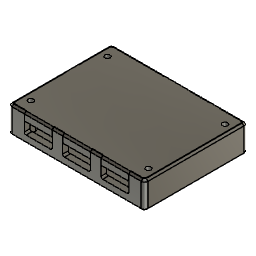
HDMI_Switcher v4 (Autodesk Fusion 360 design; units mm, degrees)
Autodesk Fusion 360 part; units mm, degrees
sketch "Sketch1" plane through (0, 0, 0) normal (0, 0, 1) x (1, 0, 0)
  line L0 (37, -29.5) -> (-37, -29.5)
  line L1 (-38.75, -27.5) -> (-38.75, 27.5)
  line L2 (-37, 29.5) -> (37, 29.5)
  line L3 (38.75, 27.5) -> (38.75, -27.5)
  line L4 (38.75, -29.5) -> (-38.75, 29.5) construction
  line L5 (-38.75, -29.5) -> (38.75, 29.5) construction
  line L6 (36, -28.5) -> (-36, -28.5)
  line L7 (-37.75, -26.5) -> (-37.75, 26.5)
  line L8 (-36, 28.5) -> (36, 28.5)
  line L9 (37.75, 26.5) -> (37.75, -26.5)
  line L10 (37.75, -28.5) -> (-37.75, 28.5) construction
  line L11 (-37.75, -28.5) -> (37.75, 28.5) construction
  arc A0 (-36.75, 29.5) -> (-38.75, 27.5) centre (-36.75, 27.5) ccw
  arc A1 (-35.75, 28.5) -> (-37.75, 26.5) centre (-35.75, 26.5) ccw
  arc A2 (38.75, 27.5) -> (36.75, 29.5) centre (36.75, 27.5) ccw
  arc A3 (37.75, 26.5) -> (35.75, 28.5) centre (35.75, 26.5) ccw
  arc A4 (36.75, -29.5) -> (38.75, -27.5) centre (36.75, -27.5) ccw
  arc A5 (35.75, -28.5) -> (37.75, -26.5) centre (35.75, -26.5) ccw
  arc A6 (-38.75, -27.5) -> (-36.75, -29.5) centre (-36.75, -27.5) ccw
  arc A7 (-37.75, -26.5) -> (-35.75, -28.5) centre (-35.75, -26.5) ccw
  line L12 (38.75, 26) -> (-38.75, 26)
  line L13 (-38.75, -26) -> (38.75, -26)
  line L14 (-38.75, 11.529) -> (-37.75, 11.2315) construction
  line L15 (37.75, -11.2315) -> (38.75, -11.529) construction
  line L16 (38.75, 11.529) -> (37.75, 11.2315) construction
  line L17 (-37.75, -11.2315) -> (-38.75, -11.529) construction
  line L18 (-37.75, 22.1895) -> (-33.75, 22.1895)
  line L19 (-33.75, 22.1895) -> (-33.75, -35)
  line L20 (-33.75, -26) -> (-33.75, -15)
  circle A8 centre (-33.75, -15) radius 2
  line L21 (-33.75, -15) -> (-33.75, -8.8)
  line L22 (-33.75, -15) -> (-33.75, -2)
  circle A9 centre (-33.75, -8.8) radius 2
  circle A10 centre (-33.75, -2) radius 2
  line L23 (-37.75, 24.2353) -> (-33.15, 24.2353)
  line L24 (-33.15, 24.2353) -> (-33.15, 26)
  line L25 (-33.15, 26) -> (-33.15, 15)
  circle A11 centre (-33.15, 15) radius 2
  line L26 (-33.75, 26) -> (-33.75, 22)
  circle A12 centre (-33.75, 22) radius 2.5
  line L27 (37.75, 26) -> (33.75, 26)
  line L28 (33.75, 26) -> (33.75, 22)
  line L29 (33.75, 22) -> (37.75, 22)
  line L30 (37.75, 22) -> (37.75, 26)
  circle A13 centre (33.75, 22) radius 2.5
  line L31 (37.75, -26) -> (33.75, -26)
  line L32 (33.75, -26) -> (33.75, -22)
  line L33 (33.75, -22) -> (37.75, -22)
  line L34 (37.75, -22) -> (37.75, -26)
  circle A14 centre (33.75, -22) radius 2.5
  line L35 (-37.75, -26) -> (-33.75, -26)
  line L36 (-33.75, -26) -> (-33.75, -22)
  line L37 (-33.75, -22) -> (-37.75, -22)
  line L38 (-37.75, -22) -> (-37.75, -26)
  circle A15 centre (-33.75, -22) radius 2.5
  line L39 (0, -26) -> (8, -26)
  line L40 (8, -26) -> (8, -29.5)
  line L41 (0, -26) -> (-8, -26)
  line L42 (-8, -26) -> (-8, -29.5)
  line L43 (0, 26) -> (8, 26)
  line L44 (8, 26) -> (8, 29.5)
  line L45 (0, 28.5) -> (-8, 28.5)
  line L46 (-8, 28.5) -> (-8, 29.5)
  line L47 (8, -26) -> (30, -26)
  line L48 (30, -26) -> (14, -26)
  line L49 (14, -26) -> (14, -29.5)
  line L50 (30, -26) -> (30, -29.5)
  line L51 (-8, -26) -> (-30, -26)
  line L52 (-30, -26) -> (-30, -29.5)
  line L53 (-30, -26) -> (-14, -26)
  line L54 (-14, -26) -> (-14, -29.5)
  line L55 (-39, -27.5) -> (-39, 27.5)
  arc A16 (-37, 29.5) -> (-39, 27.5) centre (-37, 27.5) ccw
  line L56 (-38, -26.5) -> (-38, 26.5)
  arc A17 (-36, 28.5) -> (-38, 26.5) centre (-36, 26.5) ccw
  arc A18 (-38, -26.5) -> (-36, -28.5) centre (-36, -26.5) ccw
  arc A19 (-39, -27.5) -> (-37, -29.5) centre (-37, -27.5) ccw
  line L57 (38, 26.5) -> (38, -26.5)
  line L58 (39, 27.5) -> (39, -27.5)
  arc A20 (38, 26.5) -> (36, 28.5) centre (36, 26.5) ccw
  arc A21 (39, 27.5) -> (37, 29.5) centre (37, 27.5) ccw
  arc A22 (36, -28.5) -> (38, -26.5) centre (36, -26.5) ccw
  arc A23 (37, -29.5) -> (39, -27.5) centre (37, -27.5) ccw
  line L59 (-8, 28.5) -> (-8, 26)
  line L60 (-8, 26) -> (-10, 26)
  line L61 (-10, 26) -> (-10, 26.25)
  line L62 (-10, 26.25) -> (-8, 26.25)
  line L63 (-10, 26.25) -> (-10, 28.5)
  line L64 (8, 26) -> (8, 26.25)
  line L65 (8, 26.25) -> (10, 26.25)
  line L66 (10, 26.25) -> (10, 28.5)
  line L67 (-8, -26) -> (-8, -26.25)
  line L68 (-8, -26.25) -> (-32, -26.25)
  line L69 (-32, -26.25) -> (31.5597, -26.25)
  line L70 (-30, -26.25) -> (-32, -26.25)
  line L71 (-32, -26.25) -> (-32, -28.5)
  line L72 (-14, -26.25) -> (-12, -26.25)
  line L73 (-12, -26.25) -> (-12, -28.5)
  line L74 (-8, -26.25) -> (-10, -26.25)
  line L75 (-10, -26.25) -> (-10, -28.5)
  line L76 (8, -26.25) -> (10, -26.25)
  line L77 (10, -26.25) -> (10, -28.5)
  line L78 (14, -26.25) -> (12, -26.25)
  line L79 (12, -26.25) -> (12, -28.5)
  line L80 (30, -26.25) -> (32, -26.25)
  line L81 (32, -26.25) -> (32, -28.5)
  line L82 (37.75, 26) -> (24.45, 26)
  line L83 (24.45, 26) -> (24.45, 28.5)
  line L84 (24.45, 28.5) -> (18.45, 28.5)
  line L85 (18.45, 28.5) -> (18.45, 29.5)
  line L86 (24.45, 28.5) -> (24.45, 29.5)
  line L87 (-38, 26) -> (-38, 10)
  line L88 (-38, 10) -> (-38, 2)
  line L89 (-38, 2) -> (-39, 2)
  line L90 (-38, 10) -> (-39, 10)
  circle A24 centre (-33.75, 22) radius 1.75
  circle A25 centre (-33.75, -22) radius 1.75
  circle A26 centre (33.75, 22) radius 1.75
  circle A27 centre (33.75, -22) radius 1.75
  line L91 (-37.5, -26.5) -> (-37.5, 26.5)
  arc A28 (-36, 28) -> (-37.5, 26.5) centre (-36, 26.5) ccw
  line L92 (-36, 28) -> (36, 28)
  arc A29 (37.5, 26.5) -> (36, 28) centre (36, 26.5) ccw
  line L93 (37.5, 26.5) -> (37.5, -26.5)
  arc A30 (36, -28) -> (37.5, -26.5) centre (36, -26.5) ccw
  line L94 (36, -28) -> (-36, -28)
  arc A31 (-37.5, -26.5) -> (-36, -28) centre (-36, -26.5) ccw
  line L95 (18.45, 28.5) -> (18.45, 28)
  line L96 (18.45, 28) -> (18.45, 26)
  line L97 (-32, -26.25) -> (-37.5, -26.25)
  line L98 (32, -26.25) -> (37.5, -26.25)
  line L99 (37.5, -26.25) -> (38, -26.25)
  line L100 (-37.5, -26.25) -> (-38, -26.25)
  line L101 (-78, -26.25) -> (-78, -28.5)
  line L102 (-90, 28.5) -> (-98, 28.5)
  line L103 (-126, 28.5) -> (-54, 28.5)
  line L104 (-100, 26.25) -> (-100, 28.5)
  line L105 (-100, 26) -> (-100, 26.25)
  line L106 (-82, 26.25) -> (-80, 26.25)
  line L107 (-71.55, 28.5) -> (-71.55, 29.5)
  line L108 (-104, -26.25) -> (-102, -26.25)
  arc A32 (-129, -27.5) -> (-127, -29.5) centre (-127, -27.5) ccw
  line L109 (-90, 26) -> (-82, 26)
  line L110 (-98, -26.25) -> (-122, -26.25)
  circle A33 centre (-123.75, -22) radius 2.5
  line L111 (-120, -26.25) -> (-122, -26.25)
  arc A34 (-52, 26.5) -> (-54, 28.5) centre (-54, 26.5) ccw
  arc A35 (-51, 27.5) -> (-53, 29.5) centre (-53, 27.5) ccw
  arc A36 (-128, -26.5) -> (-126, -28.5) centre (-126, -26.5) ccw
  line L112 (-65.55, 28.5) -> (-65.55, 29.5)
  line L113 (-104, -26) -> (-104, -29.5)
  line L114 (-71.55, 28.5) -> (-71.55, 28)
  line L115 (-128.75, 11.529) -> (-127.75, 11.2315) construction
  line L116 (-98, -26) -> (-98, -26.25)
  line L117 (-127.5, -26.25) -> (-128, -26.25)
  line L118 (-100, 26.25) -> (-98, 26.25)
  line L119 (-51.25, 11.529) -> (-52.25, 11.2315) construction
  arc A37 (-127, 29.5) -> (-129, 27.5) centre (-127, 27.5) ccw
  line L120 (-127.75, -22) -> (-127.75, -26)
  line L121 (-98, -26.25) -> (-100, -26.25)
  line L122 (-102, -26.25) -> (-102, -28.5)
  line L123 (-60, -26) -> (-60, -29.5)
  circle A38 centre (-56.25, -22) radius 2.5
  line L124 (-51.25, 26) -> (-128.75, 26)
  line L125 (-122, -26.25) -> (-127.5, -26.25)
  line L126 (-80, 26.25) -> (-80, 28.5)
  line L127 (-65.55, 26) -> (-65.55, 28.5)
  line L128 (-128, 10) -> (-129, 10)
  line L129 (-52.25, -22) -> (-52.25, -26)
  line L130 (-120, -26) -> (-120, -29.5)
  line L131 (-82, -26.25) -> (-80, -26.25)
  line L132 (-82, 26) -> (-82, 29.5)
  line L133 (-52.5, -26.25) -> (-52, -26.25)
  line L134 (-52.25, 26) -> (-65.55, 26)
  line L135 (-98, -26) -> (-98, -29.5)
  line L136 (-60, -26.25) -> (-58, -26.25)
  line L137 (-122, -26.25) -> (-122, -28.5)
  line L138 (-65.55, 28.5) -> (-71.55, 28.5)
  circle A39 centre (-56.25, 22) radius 2.5
  circle A40 centre (-56.25, 22) radius 1.75
  line L139 (-128, 2) -> (-129, 2)
  line L140 (-98, 28.5) -> (-98, 29.5)
  line L141 (-52.25, 26) -> (-56.25, 26)
  line L142 (-100, -26.25) -> (-100, -28.5)
  line L143 (-82, -26) -> (-82, -29.5)
  line L144 (-80, -26.25) -> (-80, -28.5)
  line L145 (-98, 26) -> (-100, 26)
  line L146 (-82, 26) -> (-82, 26.25)
  line L147 (-128, 10) -> (-128, 2)
  line L148 (-52.25, 22) -> (-52.25, 26)
  line L149 (-71.55, 28) -> (-71.55, 26)
  line L150 (-98, 28.5) -> (-98, 26)
  arc A41 (-126, 28.5) -> (-128, 26.5) centre (-126, 26.5) ccw
  circle A42 centre (-123.75, -22) radius 1.75
  line L151 (-128, 26) -> (-128, 10)
  line L152 (-58, -26.25) -> (-58, -28.5)
  circle A43 centre (-123.75, 22) radius 1.75
  circle A44 centre (-123.75, 22) radius 2.5
  arc A45 (-125.75, 28.5) -> (-127.0797, 27.9939) centre (-125.75, 26.5) ccw
  line L153 (-58, -26.25) -> (-52.5, -26.25)
  line L154 (-52, 26.5) -> (-52, -26.5)
  line L155 (-76, -26) -> (-76, -29.5)
  arc A46 (-54, -28.5) -> (-52, -26.5) centre (-54, -26.5) ccw
  line L156 (-122, -26.25) -> (-58.4403, -26.25)
  arc A47 (-53, -29.5) -> (-51, -27.5) centre (-53, -27.5) ccw
  line L157 (-76, -26.25) -> (-78, -26.25)
  circle A48 centre (-56.25, -22) radius 1.75
  line L158 (-51, 27.5) -> (-51, -27.5)
  line L159 (-52.25, -11.2315) -> (-51.25, -11.529) construction
  line L160 (-128, -26.5) -> (-128, 26.5)
  line L161 (-127, 29.5) -> (-98, 29.5)
  line L162 (-98, 29.5) -> (-82, 29.5)
  line L163 (-82, 29.5) -> (-71.55, 29.5)
  line L164 (-53.25, 29.5) -> (-53, 29.5)
  line L165 (-65.55, 29.5) -> (-53.25, 29.5)
  line L166 (-71.55, 29.5) -> (-65.55, 29.5)
  line L167 (-129, -27.5) -> (-129, 2)
  line L168 (-129, 10) -> (-129, 27.5)
  line L169 (-129, 2) -> (-129, 10)
  line L170 (-120, -29.5) -> (-127, -29.5)
  line L171 (-104, -29.5) -> (-120, -29.5)
  line L172 (-120, -28.5) -> (-126, -28.5)
  line L173 (-104, -28.5) -> (-120, -28.5)
  line L174 (-98, -29.5) -> (-104, -29.5)
  line L175 (-82, -29.5) -> (-98, -29.5)
  line L176 (-98, -28.5) -> (-104, -28.5)
  line L177 (-82, -28.5) -> (-98, -28.5)
  line L178 (-53, -29.5) -> (-60, -29.5)
  line L179 (-76, -29.5) -> (-82, -29.5)
  line L180 (-60, -29.5) -> (-76, -29.5)
  line L181 (-54, -28.5) -> (-60, -28.5)
  line L182 (-76, -28.5) -> (-82, -28.5)
  line L183 (-60, -28.5) -> (-76, -28.5)
  line L184 (-127.75, 24.2353) -> (-127.5, 24.2353)
  line L185 (-127.75, 22.1895) -> (-127.5, 22.1895)
  line L186 (-123.75, 22.1895) -> (-123.75, 22)
  line L187 (-123.75, 26) -> (-123.75, 25.4801)
  arc A49 (-126, 28.25) -> (-127.75, 26.5) centre (-126, 26.5) ccw
  line L188 (-127.75, -26.5) -> (-127.75, 26.5)
  arc A50 (-127.75, -26.5) -> (-126, -28.25) centre (-126, -26.5) ccw
  line L189 (-120, -28.25) -> (-126, -28.25)
  line L190 (-104, -28.25) -> (-120, -28.25)
  line L191 (-98, -28.25) -> (-104, -28.25)
  line L192 (-82, -28.25) -> (-98, -28.25)
  line L193 (-76, -28.25) -> (-82, -28.25)
  line L194 (-60, -28.25) -> (-76, -28.25)
  line L195 (-54, -28.25) -> (-60, -28.25)
  arc A51 (-54, -28.25) -> (-52.25, -26.5) centre (-54, -26.5) ccw
  line L196 (-52.25, 26.5) -> (-52.25, -26.5)
  arc A52 (-52.25, 26.5) -> (-54, 28.25) centre (-54, 26.5) ccw
  line L197 (-126, 28.25) -> (-54, 28.25)
  line L198 (-98, 26) -> (-97.9, 26)
  line L199 (-97.9, 26) -> (-97.9, 28.25)
  line L200 (-82, 26) -> (-82.1, 26)
  line L201 (-82.1, 26) -> (-82.1, 28.25)
  line L202 (-71.55, 26) -> (-71.45, 26)
  line L203 (-71.45, 26) -> (-71.45, 28.25)
  line L204 (-65.55, 26) -> (-65.65, 26)
  line L205 (-65.65, 26) -> (-65.65, 28.25)
  line L206 (-129, 10) -> (-129, 9.9)
  line L207 (-129, 9.9) -> (-127.75, 9.9)
  line L208 (-129, 2) -> (-129, 2.1)
  line L209 (-129, 2.1) -> (-127.75, 2.1)
  line L210 (-120, -26.25) -> (-119.9, -26.25)
  line L211 (-119.9, -26.25) -> (-119.9, -29.5)
  line L212 (-104, -29.5) -> (-104.1, -29.5)
  line L213 (-104.1, -29.5) -> (-104.0981, -26.25)
  line L214 (-98, -29.5) -> (-97.9, -29.5)
  line L215 (-97.9, -29.5) -> (-97.9, -26.25)
  line L216 (-82, -29.5) -> (-82.1, -29.5)
  line L217 (-82.1, -29.5) -> (-82.1, -26.25)
  line L218 (-76, -29.5) -> (-75.9, -29.5)
  line L219 (-75.9, -29.5) -> (-75.9, -26.25)
  line L220 (-60, -29.5) -> (-60.1, -29.5)
  line L221 (-60.1, -29.5) -> (-60.1, -26.25)
  line L222 (-97.9, 28.25) -> (-97.9, 29.5)
  line L223 (-82.1, 28.25) -> (-82.1, 29.5)
  line L224 (-71.45, 28.25) -> (-71.45, 29.5)
  line L225 (-65.65, 28.25) -> (-65.65, 29.5)
  line L226 (-33.75, 24.5) -> (-37.5, 24.5)
  line L227 (-33.75, 19.5) -> (-37.5, 19.5)
  line L228 (33.75, 24.5) -> (37.5, 24.5)
  line L229 (33.75, 19.5) -> (37.5, 19.5)
  line L230 (33.75, -24.5) -> (37.5, -24.5)
  line L231 (33.75, -19.5) -> (37.5, -19.5)
  line L232 (-33.75, -19.5) -> (-37.5, -19.5)
  line L233 (-33.75, -24.5) -> (-37.5, -24.5)
  line L234 (-31.25, 22) -> (-31.25, 26)
  line L235 (31.25, 22) -> (31.25, 26.5)
  line L236 (31.25, -22) -> (31.25, -27)
  line L237 (-31.25, -22) -> (-31.25, -27)
  circle A53 centre (-56.25, 22) radius 1.5
  circle A54 centre (-123.75, -22) radius 1.5
  circle A55 centre (-56.25, -22) radius 1.5
  circle A56 centre (-123.75, 22) radius 1.5
  line L238 (-38, 10) -> (-37.5, 10)
  line L239 (-38, 2) -> (-37.5, 2)
  point P0 (-90, 0)
  point P1 (-90, 0)
  point P2 (-90, 0)
  dimension "d1" = 77.5
  dimension "d2" = 59
  dimension "d3" = 75.5
  dimension "d4" = 57
  dimension "d5" = 2
  dimension "d6" = 2
  dimension "d8" = 4
  dimension "d9" = 11
  dimension "d10" = 4
  dimension "d11" = 6.2
  dimension "d12" = 13
  dimension "d13" = 4
  dimension "d14" = 4
  dimension "d15" = 4.6
  dimension "d16" = 11
  dimension "d17" = 4
  dimension "d19" = 4
  dimension "d20" = 5
  dimension "d21" = 4
  dimension "d22" = 4
  dimension "d23" = 5
  dimension "d24" = 4
  dimension "d25" = 4
  dimension "d26" = 5
  dimension "d27" = 4
  dimension "d28" = 4
  dimension "d29" = 5
  dimension "d32" = 8
  dimension "d33" = 8
  dimension "d34" = 8
  dimension "d35" = 8
  dimension "d36" = 22
  dimension "d37" = 16
  dimension "d38" = 22
  dimension "d39" = 16
  dimension "d41" = 2
  dimension "d43" = 2
  dimension "d46" = 2
  dimension "d47" = 2
  dimension "d48" = 0.25
  dimension "d49" = 0.25
  dimension "d50" = 2
  dimension "d51" = 0.25
  dimension "d52" = 2
  dimension "d53" = 2
  dimension "d54" = 2
  dimension "d55" = 2
  dimension "d56" = 2
  dimension "d57" = 2
  dimension "d58" = 13.3
  dimension "d59" = 6
  dimension "d62" = 16
  dimension "d63" = 8
  dimension "d72" = 3.5
  dimension "d73" = 3.5
  dimension "d74" = 3.5
  dimension "d75" = 3.5
  dimension "d80" = -0.5
  dimension "d102" = 4
  dimension "d103" = 4
  dimension "d104" = 5
  dimension "d106" = 4
  dimension "d107" = 5
  dimension "d109" = 4
  dimension "d110" = 5
  dimension "d113" = 8
  dimension "d114" = 8
  dimension "d115" = 22
  dimension "d116" = 16
  dimension "d117" = 22
  dimension "d118" = 16
  dimension "d124" = 2
  dimension "d126" = 2
  dimension "d127" = 0.25
  dimension "d128" = 0.25
  dimension "d129" = 2
  dimension "d130" = 0.25
  dimension "d131" = 2
  dimension "d132" = 2
  dimension "d133" = 2
  dimension "d134" = 2
  dimension "d135" = 2
  dimension "d136" = 2
  dimension "d137" = 13.3
  dimension "d138" = 6
  dimension "d139" = 16
  dimension "d140" = 8
  dimension "d142" = 3.5
  dimension "d143" = 3.5
  dimension "d144" = 3.5
  dimension "d145" = 0.25
  dimension "d146" = 0.1
  dimension "d147" = 0.1
  dimension "d148" = 0.1
  dimension "d149" = 0.1
  dimension "d150" = 0.1
  dimension "d151" = 0.1
  dimension "d152" = 0.1
  dimension "d153" = 0.1
  dimension "d154" = 0.1
  dimension "d155" = 0.1
  dimension "d156" = 0.1
  dimension "d157" = 0.1
  dimension "d174" = 3
  dimension "d176" = 3
  dimension "d177" = 3
  dimension "d178" = 3
  constraint horizontal L0
  constraint perpendicular L0 L1
  constraint parallel L0 L2
  constraint parallel L1 L3
  constraint coincident L4 origin
  constraint coincident L5 origin
  constraint horizontal L6
  constraint perpendicular L6 L7
  constraint parallel L6 L8
  constraint parallel L7 L9
  constraint coincident L10 origin
  constraint coincident L11 origin
  constraint coincident L4.end L1
  constraint coincident L4.end L2
  constraint tangent L1 A0
  constraint tangent L2 A0
  constraint coincident L10.end L8
  constraint coincident L10.end L7
  constraint tangent L8 A1
  constraint tangent L7 A1
  constraint coincident L5.end L2
  constraint coincident L5.end L3
  constraint tangent L2 A2
  constraint tangent L3 A2
  constraint equal A1 A2
  constraint coincident L11.end L8
  constraint coincident L11.end L9
  constraint tangent L8 A3
  constraint tangent L9 A3
  constraint equal A1 A3
  constraint coincident L4.start L0
  constraint coincident L4.start L3
  constraint tangent L0 A4
  constraint tangent L3 A4
  constraint equal A1 A4
  constraint coincident L10.start L9
  constraint coincident L10.start L6
  constraint tangent L9 A5
  constraint tangent L6 A5
  constraint equal A1 A5
  constraint coincident L5.start L0
  constraint coincident L5.start L1
  constraint tangent L0 A6
  constraint tangent L1 A6
  constraint equal A1 A6
  constraint coincident L11.start L7
  constraint coincident L11.start L6
  constraint tangent L7 A7
  constraint tangent L6 A7
  constraint equal A1 A7
  constraint horizontal L12
  constraint parallel L12 L13
  constraint coincident origin L16
  constraint coincident origin L14
  constraint coincident L1 L12.end
  constraint coincident L1 L13.start
  constraint coincident L1 L17.end
  constraint coincident L1 L14.start
  constraint coincident L3 L15.end
  constraint coincident L3 L16.start
  constraint coincident L3 L12.start
  constraint coincident L3 L13.end
  constraint coincident L9 L15.start
  constraint collinear L14 L15
  constraint coincident L9 L16.end
  constraint collinear L16 L17
  constraint coincident L7 L14.end
  constraint coincident L7 L17.start
  constraint coincident L7 L18.start
  constraint perpendicular L7 L18
  constraint perpendicular L0 L19
  constraint coincident L19 L20.start
  constraint coincident L13 L20.start
  constraint perpendicular L13 L20
  constraint coincident L20.end A8.centre
  constraint parallel L19 L21
  constraint parallel L21 L22
  constraint coincident L21.end A9.centre
  constraint coincident L22.end A10.centre
  constraint coincident L7 L23.start
  constraint perpendicular L7 L23
  constraint coincident L12 L24.end
  constraint perpendicular L12 L24
  constraint perpendicular L23 L25
  constraint coincident L25.end A11.centre
  constraint coincident L12 L26.start
  constraint perpendicular L23 L26
  constraint coincident L26.end A12.centre
  constraint horizontal L27
  constraint vertical L28
  constraint horizontal L29
  constraint vertical L30
  constraint coincident L9 L27.start
  constraint coincident L12 L27.start
  constraint coincident L28.end L29.start
  constraint horizontal L31
  constraint vertical L32
  constraint horizontal L33
  constraint vertical L34
  constraint coincident L9 L31.start
  constraint coincident L13 L31.start
  constraint coincident L32.end L33.start
  constraint horizontal L35
  constraint vertical L36
  constraint horizontal L37
  constraint vertical L38
  constraint coincident L7 L35.start
  constraint coincident L13 L35.start
  constraint coincident L36.end L37.start
  constraint midpoint L13 L39.start
  constraint parallel L13 L39
  constraint coincident L0 L40.end
  constraint perpendicular L0 L40
  constraint perpendicular L40 L41
  constraint coincident L0 L42.end
  constraint perpendicular L0 L42
  constraint midpoint L12 L43.start
  constraint perpendicular L3 L43
  constraint coincident L2 L44.end
  constraint perpendicular L2 L44
  constraint perpendicular L44 L45
  constraint coincident L2 L46.end
  constraint perpendicular L2 L46
  constraint perpendicular L40 L47
  constraint coincident L47 L48.end
  constraint coincident L0 L49.end
  constraint perpendicular L0 L49
  constraint coincident L0 L50.end
  constraint perpendicular L0 L50
  constraint perpendicular L42 L51
  constraint coincident L0 L52.end
  constraint perpendicular L0 L52
  constraint perpendicular L52 L53
  constraint coincident L0 L54.end
  constraint perpendicular L0 L54
  constraint coincident L2 A0.start
  constraint tangent L2 A16
  constraint tangent L55 A16
  constraint coincident L8 L45.start
  constraint coincident L8 A1.start
  constraint tangent L8 A17
  constraint tangent L56 A17
  constraint coincident L6 A7.end
  constraint tangent L6 A18
  constraint tangent L56 A18
  constraint equal A17 A18
  constraint coincident L0 A6.end
  constraint tangent L0 A19
  constraint tangent L55 A19
  constraint equal A17 A19
  constraint coincident L8 A3.end
  constraint tangent L8 A20
  constraint tangent L57 A20
  constraint coincident L2 A2.end
  constraint tangent L58 A21
  constraint tangent L2 A21
  constraint equal A20 A21
  constraint coincident L6 A5.start
  constraint tangent L57 A22
  constraint tangent L6 A22
  constraint equal A20 A22
  constraint coincident L0 A4.start
  constraint tangent L58 A23
  constraint tangent L0 A23
  constraint equal A20 A23
  constraint coincident L12 L59.end
  constraint perpendicular L12 L59
  constraint coincident L12 L60.end
  constraint perpendicular L60 L61
  constraint coincident L59 L62.end
  constraint perpendicular L59 L62
  constraint coincident L8 L63.end
  constraint perpendicular L8 L63
  constraint vertical L64
  constraint perpendicular L44 L65
  constraint coincident L8 L66.end
  constraint perpendicular L8 L66
  constraint vertical L67
  constraint perpendicular L52 L68
  constraint parallel L13 L69
  constraint coincident L52 L70.start
  constraint coincident L68 L70.start
  constraint perpendicular L52 L70
  constraint coincident L6 L71.end
  constraint perpendicular L6 L71
  constraint coincident L54 L72.start
  constraint coincident L68 L72.start
  constraint perpendicular L54 L72
  constraint coincident L6 L73.end
  constraint perpendicular L6 L73
  constraint perpendicular L42 L74
  constraint coincident L6 L75.end
  constraint perpendicular L6 L75
  constraint coincident L40 L76.start
  constraint coincident L69 L76.start
  constraint perpendicular L40 L76
  constraint coincident L6 L77.end
  constraint perpendicular L6 L77
  constraint coincident L49 L78.start
  constraint perpendicular L49 L78
  constraint coincident L6 L79.end
  constraint perpendicular L6 L79
  constraint coincident L50 L80.start
  constraint coincident L69 L80.start
  constraint perpendicular L50 L80
  constraint coincident L6 L81.end
  constraint perpendicular L6 L81
  constraint coincident L12 L82.end
  constraint coincident L8 L83.end
  constraint perpendicular L8 L83
  constraint coincident L8 L84.end
  constraint coincident L2 L85.end
  constraint perpendicular L2 L85
  constraint coincident L2 L86.end
  constraint perpendicular L2 L86
  constraint coincident L56 L87.start
  constraint coincident L12 L87.start
  constraint perpendicular L18 L87
  constraint parallel L7 L88
  constraint coincident L55 L89.end
  constraint perpendicular L55 L89
  constraint coincident L55 L90.end
  constraint perpendicular L55 L90
  constraint concentric A12 A24
  constraint concentric A15 A25
  constraint concentric A13 A26
  constraint concentric A14 A27
  constraint coincident L92 L95.end
  constraint perpendicular L92 L95
  constraint coincident L12 L96.end
  constraint perpendicular L12 L96
  constraint coincident L91 L97.end
  constraint perpendicular L91 L97
  constraint coincident L93 L98.end
  constraint perpendicular L93 L98
  constraint coincident L57 L99.end
  constraint perpendicular L57 L99
  constraint coincident L56 L100.end
  constraint perpendicular L56 L100
  constraint horizontal L178
  constraint parallel L161 L178
  constraint horizontal L181
  constraint parallel L103 L181
  constraint tangent L103 A45
  constraint horizontal L124
  constraint coincident P2 L119
  constraint coincident P2 L115
  constraint coincident P2 P1
  constraint collinear L115 L159
  constraint coincident L187.start L124
  constraint perpendicular L184 L187
  constraint coincident A43.centre A44.centre
  constraint horizontal L141
  constraint vertical L148
  constraint coincident L134.start L124
  constraint vertical L129
  constraint vertical L120
  constraint perpendicular L143 L178
  constraint coincident L135.end L178
  constraint perpendicular L135 L178
  constraint midpoint L109.start L124
  constraint coincident L132.end L161
  constraint perpendicular L132 L161
  constraint perpendicular L102 L132
  constraint perpendicular L140 L161
  constraint coincident L155.end L178
  constraint perpendicular L155 L178
  constraint perpendicular L123 L178
  constraint coincident L130.end L178
  constraint perpendicular L130 L178
  constraint perpendicular L113 L178
  constraint tangent A37 L161
  constraint tangent A37 L167
  constraint coincident L102.start L103
  constraint coincident A45.start L103
  constraint tangent L103 A41
  constraint tangent A41 L160
  constraint tangent A36 L181
  constraint tangent A36 L160
  constraint equal A36 A41
  constraint tangent A32 L178
  constraint tangent A32 L167
  constraint equal A32 A41
  constraint tangent L103 A34
  constraint tangent A34 L154
  constraint coincident L164.start L161
  constraint tangent A35 L158
  constraint tangent A35 L161
  constraint equal A34 A35
  constraint tangent L154 A46
  constraint tangent A46 L181
  constraint equal A34 A46
  constraint tangent A47 L158
  constraint tangent A47 L178
  constraint equal A34 A47
  constraint coincident L145.start L124
  constraint perpendicular L124 L150
  constraint coincident L105.start L124
  constraint perpendicular L105 L145
  constraint coincident L118.end L150
  constraint perpendicular L118 L150
  constraint coincident L104.end L103
  constraint perpendicular L103 L104
  constraint vertical L146
  constraint perpendicular L106 L132
  constraint coincident L126.end L103
  constraint perpendicular L103 L126
  constraint vertical L116
  constraint perpendicular L110 L130
  constraint coincident L111.start L130
  constraint coincident L111.start L110
  constraint perpendicular L111 L130
  constraint coincident L137.end L181
  constraint perpendicular L137 L181
  constraint coincident L108.start L113
  constraint coincident L108.start L110
  constraint perpendicular L108 L113
  constraint coincident L122.end L181
  constraint perpendicular L122 L181
  constraint perpendicular L121 L135
  constraint coincident L142.end L181
  constraint perpendicular L142 L181
  constraint coincident L131.start L143
  constraint coincident L131.start L156
  constraint perpendicular L131 L143
  constraint coincident L144.end L181
  constraint perpendicular L144 L181
  constraint coincident L157.start L155
  constraint perpendicular L155 L157
  constraint coincident L101.end L181
  constraint perpendicular L101 L181
  constraint coincident L136.start L123
  constraint coincident L136.start L156
  constraint perpendicular L123 L136
  constraint coincident L152.end L181
  constraint perpendicular L152 L181
  constraint coincident L127.start L124
  constraint coincident L112.start L103
  constraint perpendicular L103 L127
  constraint coincident L107.start L103
  constraint coincident L107.end L161
  constraint perpendicular L107 L161
  constraint coincident L112.end L161
  constraint perpendicular L112 L161
  constraint coincident L151.start L160
  constraint coincident L151.start L124
  constraint perpendicular L151 L185
  constraint perpendicular L139 L167
  constraint coincident L128.end L167
  constraint perpendicular L128 L167
  constraint concentric A43 A44
  constraint concentric A33 A42
  constraint concentric A39 A40
  constraint concentric A38 A48
  constraint coincident L149.end L124
  constraint perpendicular L124 L149
  constraint coincident L133.end L154
  constraint perpendicular L133 L154
  constraint coincident L117.end L160
  constraint perpendicular L117 L160
  constraint coincident L113 L173.start
  constraint coincident L130 L172.start
  constraint coincident L143 L177.start
  constraint coincident L135 L176.start
  constraint coincident L123 L181.end
  constraint coincident L155 L182.start
  constraint collinear L186 L187
  constraint perpendicular L150 L198
  constraint coincident L197 L199.end
  constraint perpendicular L197 L199
  constraint horizontal L200
  constraint coincident L197 L201.end
  constraint perpendicular L197 L201
  constraint horizontal L202
  constraint coincident L197 L203.end
  constraint perpendicular L197 L203
  constraint horizontal L204
  constraint coincident L197 L205.end
  constraint perpendicular L197 L205
  constraint vertical L206
  constraint coincident L188 L207.end
  constraint perpendicular L188 L207
  constraint vertical L208
  constraint coincident L188 L209.end
  constraint perpendicular L188 L209
  constraint horizontal L210
  constraint coincident L171 L211.end
  constraint perpendicular L171 L211
  constraint horizontal L212
  constraint coincident L110 L213.end
  constraint coincident L156 L213.end
  constraint horizontal L214
  constraint coincident L156 L215.end
  constraint perpendicular L156 L215
  constraint horizontal L216
  constraint coincident L156 L217.end
  constraint perpendicular L156 L217
  constraint horizontal L218
  constraint coincident L156 L219.end
  constraint perpendicular L156 L219
  constraint horizontal L220
  constraint coincident L156 L221.end
  constraint perpendicular L156 L221
  constraint coincident L162 L222.end
  constraint perpendicular L162 L222
  constraint coincident L162 L223.end
  constraint perpendicular L162 L223
  constraint coincident L166 L224.end
  constraint perpendicular L166 L224
  constraint coincident L166 L225.end
  constraint perpendicular L166 L225
  constraint coincident A12 L226.start
  constraint coincident L26 L226.start
  constraint coincident L91 L226.end
  constraint tangent A12 L226
  constraint coincident A12 L227.start
  constraint coincident L19 L227.start
  constraint coincident L91 L227.end
  constraint tangent A12 L227
  constraint perpendicular L91 L227
  constraint coincident A13 L228.start
  constraint coincident L28 L228.start
  constraint coincident L93 L228.end
  constraint tangent A13 L228
  constraint coincident A13 L229.start
  constraint coincident L93 L229.end
  constraint tangent A13 L229
  constraint perpendicular L9 L229
  constraint coincident A14 L230.start
  constraint coincident L32 L230.start
  constraint coincident L93 L230.end
  constraint tangent A14 L230
  constraint coincident A14 L231.start
  constraint coincident L93 L231.end
  constraint tangent A14 L231
  constraint perpendicular L93 L231
  constraint coincident A15 L232.start
  constraint coincident L20 L232.start
  constraint coincident L91 L232.end
  constraint tangent A15 L232
  constraint coincident A15 L233.start
  constraint coincident L36 L233.start
  constraint coincident L91 L233.end
  constraint tangent A15 L233
  constraint coincident A12 L234.start
  constraint coincident L12 L234.end
  constraint tangent A12 L234
  constraint perpendicular L12 L234
  constraint coincident A13 L235.start
  constraint tangent A13 L235
  constraint perpendicular L82 L235
  constraint coincident A14 L236.start
  constraint tangent A14 L236
  constraint perpendicular L80 L236
  constraint coincident A15 L237.start
  constraint tangent A15 L237
  constraint perpendicular L68 L237
  constraint concentric A40 A53
  constraint concentric A33 A54
  constraint concentric A38 A55
  constraint concentric A43 A56
  constraint coincident L91 L238.end
  constraint perpendicular L91 L238
  constraint coincident L91 L239.end
  constraint perpendicular L91 L239
  measures "d1" distance of L4.end L5.end
  measures "d2" distance of L5.start L4.end
  measures "d3" distance of L10.end L11.end
  measures "d4" distance of L11.start L10.end
  measures "d5" radius of A0
  measures "d6" radius of A1
  measures "d8" distance of L18.start L18.end
  measures "d9" distance of L20.start L20.end
  measures "d10" diameter of A8
  measures "d11" distance of L20.end L21.end
  measures "d12" distance of L20.end L22.end
  measures "d13" diameter of A9
  measures "d14" diameter of A10
  measures "d15" distance of L23.start L23.end
  measures "d16" distance of L24.end L25.end
  measures "d17" diameter of A11
  measures "d19" distance of L26.start L26.end
  measures "d20" diameter of A12
  measures "d21" distance of L27.start L27.end
  measures "d22" distance of L27.start L29.end
  measures "d23" diameter of A13
  measures "d24" distance of L31.start L31.end
  measures "d25" distance of L31.start L33.end
  measures "d26" diameter of A14
  measures "d27" distance of L35.start L20.start
  measures "d28" distance of L35.start L37.end
  measures "d29" diameter of A15
  measures "d32" distance of L39.start L39.end
  measures "d33" distance of L39.start L41.end
  measures "d34" distance of L43.start L43.end
  measures "d35" distance of L45.start L45.end
  measures "d36" distance of L39.end L47.end
  measures "d37" distance of L47.end L48.end
  measures "d38" distance of L41.end L51.end
  measures "d39" distance of L51.end L53.end
  measures "d41" radius of A16
  measures "d43" radius of A17
  measures "d46" radius of A20
  measures "d47" distance of L59.end L60.end
  measures "d48" distance of L60.end L61.end
  measures "d49" distance of L43.end L64.end
  measures "d50" distance of L64.end L65.end
  measures "d51" distance of L41.end L67.end
  measures "d52" distance of L70.start L68.end
  measures "d53" distance of L72.start L72.end
  measures "d54" distance of L67.end L74.end
  measures "d55" distance of L76.start L76.end
  measures "d56" distance of L78.start L78.end
  measures "d57" distance of L80.start L80.end
  measures "d58" distance of L27.start L82.end
  measures "d59" distance of L83.end L84.end
  measures "d62" distance of L87.start L87.end
  measures "d63" distance of L87.end L88.end
  measures "d72" diameter of A24
  measures "d73" diameter of A25
  measures "d74" diameter of A26
  measures "d75" diameter of A27
  measures "d102" distance of L134.start L141.end
  measures "d103" distance of L134.start L148.start
  measures "d104" diameter of A39
  measures "d106" distance of L129.start L129.end
  measures "d107" diameter of A38
  measures "d109" distance of L120.end L120.start
  measures "d110" diameter of A33
  measures "d113" distance of L109.start L109.end
  measures "d114" distance of L102.end L102.start
  measures "d115" distance of L123.start L143.start
  measures "d116" distance of L155.start L123.start
  measures "d117" distance of L130.start L116.start
  measures "d118" distance of L113.start L130.start
  measures "d124" radius of A34
  measures "d126" distance of L105.start L145.start
  measures "d127" distance of L105.start L104.start
  measures "d128" distance of L106.start L109.end
  measures "d129" distance of L106.start L106.end
  measures "d130" distance of L110.start L116.start
  measures "d131" distance of L110.end L111.start
  measures "d132" distance of L108.end L108.start
  measures "d133" distance of L110.start L121.end
  measures "d134" distance of L131.start L131.end
  measures "d135" distance of L157.start L101.start
  measures "d136" distance of L136.start L136.end
  measures "d137" distance of L134.start L127.start
  measures "d138" distance of L112.start L107.start
  measures "d139" distance of L151.start L128.start
  measures "d140" distance of L139.start L128.start
  measures "d142" diameter of A42
  measures "d143" diameter of A40
  measures "d144" diameter of A48
  measures "d146" distance of L145.start L198.end
  measures "d147" distance of L109.end L200.end
  measures "d148" distance of L149.end L202.end
  measures "d149" distance of L127.start L204.end
  measures "d150" distance of L128.end L206.end
  measures "d151" distance of L139.end L208.end
  measures "d152" distance of L111.start L210.end
  measures "d153" distance of L113.end L212.end
  measures "d154" distance of L135.end L214.end
  measures "d155" distance of L143.end L216.end
  measures "d156" distance of L155.end L218.end
  measures "d157" distance of L123.end L220.end
  measures "d174" diameter of A53
  measures "d176" diameter of A54
  measures "d177" diameter of A55
  measures "d178" diameter of A56
extrude "Extrude1" add sketch "Sketch1" against normal blind 1 contours L0 L2 L3 A2 A4 L58 A21 A23 | L0 L3 L6 A4 L13 L50 L57 A22 | L0 L6 L49 L50 | L0 L6 L40 L49 | L6 L50 L81 L94 | L6 L49 L50 L94 | L3 L12 L13 L57 | L0 L6 L40 L42 | L6 L49 L79 L94 | L6 L9 A5 L81 L93 A30 L94 L99 | L49 L50 L69 L94 | L50 L69 L80 L81 L94 | L2 L3 L8 A2 L12 L57 A20 L86 | L9 L13 L57 L99 | L9 L12 L13 L30 L34 L57 | L0 L6 L42 L54 | L6 L40 L77 L94 | L6 L40 L42 L94 | L6 L77 L79 L94 | L49 L69 L78 L79 L94 | L6 L9 A5 L57 A22 L99 | L81 L93 A30 L94 L98 | L13 L47 L48 L49 L50 L69 | L13 L50 L69 L80 L236 | L8 L9 A3 L12 L57 A20 | L9 L13 L31 L33 L34 L93 | L9 L13 L31 L93 L99 | L2 L8 L84 L85 L86 | L0 L6 L52 L54 | L6 L42 L75 L94 | L40 L42 L69 L94 | L40 L69 L76 L77 L94 | L69 L77 L79 L94 | L13 L40 L47 L49 L69 L76 L78 | L13 L31 L69 L80 L93 L98 L236 | L12 L13 L19 L20 A8 L21 L22 A9 A10 L25 A11 A12 A13 A14 A15 L39 L41 L43 L47 L48 L51 L53 L60 L82 L93 L229 L231 L234 L235 L236 L237 | L8 L9 A3 L12 L27 L82 L83 L92 A29 L93 | L9 L12 L27 L29 L30 L82 L93 | L9 L29 L33 L93 | L13 L31 L32 L93 L230 | L2 L8 L44 L85 | L8 L83 L84 L92 L95 | L0 L6 L19 L52 | L6 L54 L73 L94 | L6 L52 L54 L94 | L6 L73 L75 L94 | L42 L68 L69 L74 L75 L94 | L13 L39 L40 L41 L42 L67 L69 | L13 L32 A14 L236 | L12 L27 L28 L82 L93 L228 | L12 L27 L82 L83 L92 A29 L93 | L33 A14 L93 L230 | L33 A14 L93 L231 | L2 L8 L44 L45 L46 | L8 L66 L92 L95 | L12 L83 L92 L96 | L0 L1 L6 A6 L13 L19 L56 A18 | L6 L52 L71 L94 | L52 L54 L68 L69 L94 | L54 L68 L69 L72 L73 L94 | L68 L69 L73 L75 L94 | L13 L42 L51 L54 L67 L68 L69 L72 L74 | L32 L33 A14 A27 | L29 A13 L93 L229 | L29 A13 L93 L228 | L12 L28 A13 L82 L235 | L32 L33 A14 A27 | L1 L2 L8 A0 L12 L46 L56 A17 | L8 L44 L45 L59 L92 | L8 L44 L66 L92 | L12 L44 L64 L65 L66 L92 L96 | L0 L1 A6 L55 A19 L89 | L6 L19 L71 L94 | L6 L7 A7 L19 L91 L94 A31 L100 | L52 L68 L69 L70 L71 L94 | L13 L51 L52 L53 L54 L68 L69 | L28 L29 A13 A26 | L28 L29 A13 A26 | L32 L33 A27 | L32 L33 A27 | L1 L2 A0 L55 A16 L90 | L8 L59 L63 L92 | L44 L65 L66 L92 | L12 L43 L44 L59 L64 L92 | L6 L7 A7 L56 A18 L100 | L19 L91 L94 A31 L97 | L19 L71 L94 L97 | L13 L52 L68 L69 L70 L237 | L28 L29 A26 | L28 L29 A26 | L7 L8 A1 L12 L63 L91 A28 L92 | L59 L62 L63 L92 | L1 L13 L56 L89 | L13 L19 L35 L91 L97 | L13 L19 L68 L69 L70 L97 L237 | L1 L12 L56 L87 L90 | L7 L8 A1 L12 L56 A17 | L12 L61 L63 L91 A28 L92 | L12 L59 L60 L61 L62 | L1 L55 L89 L90 | L1 L56 L88 L89 L90 | L7 L13 L38 L56 L239 | L7 L13 L56 L100 | L7 L13 L35 L91 L100 | L13 L19 L20 L36 A15 L237 | L13 L19 L20 L35 L36 L91 L233 | L7 L12 L56 L87 L238 | L7 L56 L88 L238 L239 | L7 L13 L35 L37 L38 L91 | L19 L20 L36 L37 A15 A25 | L19 L20 L36 A15 A25 | L37 A15 L91 L233 | L7 L12 L23 L91 | L7 L37 L91 L239 | L7 L91 L238 L239 | L19 L20 L36 L37 A25 | L19 L20 L36 A25 | L19 L20 L37 A15 A25 | L37 A15 L91 L232 | L19 L20 A8 L21 L22 A9 A10 A11 L91 L227 L232 | L7 L18 L91 L238 | L7 L18 L23 L91 | L12 L26 L91 L226 | L12 L24 L25 A12 L234 | L19 L20 L37 A25 | L23 A12 L91 L226 | L18 L23 A12 L91 | L12 L24 L25 L26 A12 | L24 L25 A12 A24 | L18 A12 L91 L227 | L23 L26 A12 | L18 L23 L26 A12 A24 | L23 L24 L25 L26 A12 | L19 L25 A12 A24 | L19 L25 A11 A12 | L18 L19 A12 A24 | L23 L25 L26 A24 | L19 L25 L26 A24 | L25 A24 | L18 L26 A24 | L18 L19 L26 A24 makes body 1
extrude "Extrude2" add sketch "Sketch1" along normal blind 14.5 contours L0 L2 L3 A2 A4 L58 A21 A23 | L0 L3 L6 A4 L13 L50 L57 A22 | L0 L6 L40 L49 | L3 L12 L13 L57 | L2 L3 L8 A2 L12 L57 A20 L86 | L0 L6 L42 L54 | L2 L8 L44 L85 | L0 L6 L19 L52 | L0 L1 L6 A6 L13 L19 L56 A18 | L1 L2 L8 A0 L12 L46 L56 A17 | L0 L1 A6 L55 A19 L89 | L1 L2 A0 L55 A16 L90 | L1 L13 L56 L89 | L1 L12 L56 L87 L90 bodies 1
extrude "Extrude3" add sketch "Sketch1" along normal blind 1.5 contours L2 L8 L84 L85 L86 | L8 L83 L84 L92 L95 | L12 L83 L92 L96 bodies 1
extrude "Extrude4" add sketch "Sketch1" along normal blind 9.5 contours L13 L31 L69 L80 L93 L98 L236 | L13 L31 L32 L93 L230 | L13 L32 A14 L236 | L12 L27 L28 L82 L93 L228 | L33 A14 L93 L230 | L33 A14 L93 L231 | L32 L33 A14 A27 | L29 A13 L93 L229 | L29 A13 L93 L228 | L12 L28 A13 L82 L235 | L32 L33 A14 A27 | L28 L29 A13 A26 | L28 L29 A13 A26 | L32 L33 A27 | L32 L33 A27 | L28 L29 A26 | L28 L29 A26 | L13 L19 L35 L91 L97 | L13 L19 L68 L69 L70 L97 L237 | L13 L19 L20 L36 A15 L237 | L13 L19 L20 L35 L36 L91 L233 | L19 L20 L36 L37 A15 A25 | L19 L20 L36 A15 A25 | L37 A15 L91 L233 | L19 L20 L36 L37 A25 | L19 L20 L36 A25 | L19 L20 L37 A15 A25 | L37 A15 L91 L232 | L12 L26 L91 L226 | L12 L24 L25 A12 L234 | L19 L20 L37 A25 | L23 A12 L91 L226 | L18 L23 A12 L91 | L12 L24 L25 L26 A12 | L24 L25 A12 A24 | L18 A12 L91 L227 | L23 L26 A12 | L18 L23 L26 A12 A24 | L23 L24 L25 L26 A12 | L19 L25 A12 A24 | L18 L19 A12 A24 | L23 L25 L26 A24 | L19 L25 L26 A24 | L25 A24 | L18 L26 A24 | L18 L19 L26 A24 bodies 1
extrude "Extrude5" add sketch "Sketch1" along normal blind 2.5 contours L0 L6 L49 L50 | L6 L49 L50 L94 | L0 L6 L40 L42 | L49 L50 L69 L94 | L6 L40 L42 L94 | L13 L47 L48 L49 L50 L69 | L0 L6 L52 L54 | L40 L42 L69 L94 | L6 L52 L54 L94 | L13 L39 L40 L41 L42 L67 L69 | L2 L8 L44 L45 L46 | L52 L54 L68 L69 L94 | L8 L44 L45 L59 L92 | L13 L51 L52 L53 L54 L68 L69 | L12 L43 L44 L59 L64 L92 bodies 1
extrude "Extrude6" add sketch "Sketch1" along normal blind 13 contours L6 L50 L81 L94 | L6 L49 L79 L94 | L6 L9 A5 L81 L93 A30 L94 L99 | L50 L69 L80 L81 L94 | L6 L40 L77 L94 | L6 L77 L79 L94 | L49 L69 L78 L79 L94 | L6 L9 A5 L57 A22 L99 | L81 L93 A30 L94 L98 | L8 L9 A3 L12 L57 A20 | L6 L42 L75 L94 | L40 L69 L76 L77 L94 | L69 L77 L79 L94 | L8 L9 A3 L12 L27 L82 L83 L92 A29 L93 | L6 L54 L73 L94 | L6 L73 L75 L94 | L42 L68 L69 L74 L75 L94 | L12 L27 L82 L83 L92 A29 L93 | L8 L66 L92 L95 | L6 L52 L71 L94 | L54 L68 L69 L72 L73 L94 | L68 L69 L73 L75 L94 | L8 L44 L66 L92 | L12 L44 L64 L65 L66 L92 L96 | L6 L19 L71 L94 | L6 L7 A7 L19 L91 L94 A31 L100 | L52 L68 L69 L70 L71 L94 | L8 L59 L63 L92 | L44 L65 L66 L92 | L6 L7 A7 L56 A18 L100 | L19 L91 L94 A31 L97 | L19 L71 L94 L97 | L7 L8 A1 L12 L63 L91 A28 L92 | L59 L62 L63 L92 | L7 L8 A1 L12 L56 A17 | L12 L61 L63 L91 A28 L92 | L12 L59 L60 L61 L62 bodies 1
extrude "Extrude7" add sketch "Sketch1" along normal blind 10.5 contours L32 L33 A27 | L32 L33 A27 | L28 L29 A26 | L28 L29 A26 | L19 L20 L36 L37 A25 | L19 L20 L36 A25 | L19 L20 L37 A25 | L19 L25 L26 A24 | L25 A24 | L18 L26 A24 | L18 L19 L26 A24 bodies 1
extrude "Extrude8" add 1 faces at (-15.9167, -0.6667, 0) along direction (0, 0, 1) blind 0.5 on bodies 1 bodies 1
extrude "Extrude9" add sketch "Sketch1" along normal blind 9.5 contours L6 L50 L81 L94 | L6 L49 L79 L94 | L6 L9 A5 L81 L93 A30 L94 L99 | L9 L13 L57 L99 | L9 L12 L13 L30 L34 L57 | L6 L40 L77 L94 | L6 L77 L79 L94 | L6 L9 A5 L57 A22 L99 | L8 L9 A3 L12 L57 A20 | L9 L13 L31 L33 L34 L93 | L9 L13 L31 L93 L99 | L6 L42 L75 L94 | L8 L9 A3 L12 L27 L82 L83 L92 A29 L93 | L9 L12 L27 L29 L30 L82 L93 | L9 L29 L33 L93 | L6 L54 L73 L94 | L6 L73 L75 L94 | L8 L66 L92 L95 | L6 L52 L71 L94 | L8 L44 L66 L92 | L6 L19 L71 L94 | L6 L7 A7 L19 L91 L94 A31 L100 | L8 L59 L63 L92 | L6 L7 A7 L56 A18 L100 | L7 L8 A1 L12 L63 L91 A28 L92 | L7 L8 A1 L12 L56 A17 | L7 L13 L38 L56 L239 | L7 L13 L56 L100 | L7 L13 L35 L91 L100 | L7 L12 L56 L87 L238 | L7 L13 L35 L37 L38 L91 | L7 L12 L23 L91 | L7 L37 L91 L239 | L7 L18 L91 L238 | L7 L18 L23 L91 bodies 1
extrude "Extrude10" add sketch "Sketch1" along normal blind 1.5 separate body contours L101 L155 L156 L157 L193 | L101 L144 L156 L193 | L108 L109 L110 L111 L117 L120 L121 L124 L125 L129 L131 L133 L134 L136 L141 L145 L148 L153 L156 L157 L188 L196 L198 L200 L202 L204 L210 | L131 L143 L144 L156 L193 | L155 L156 L194 L219 | L143 L156 L192 L217 | L156 L194 L219 L221 | L183 L194 L219 L221 | L156 L192 L215 L217 | L123 L156 L194 L221 | L180 L183 L219 L221 | L177 L192 L215 L217 | L135 L156 L192 L215 | L123 L136 L152 L156 L195 | L175 L177 L215 L217 | L110 L121 L135 L142 L156 L191 | L133 L152 L153 L195 A51 L196 | L110 L122 L142 L156 L191 | L108 L110 L113 L122 L156 L191 | L110 L113 L156 L190 L213 | L110 L156 L190 L211 L213 | L171 L173 L211 L213 | L173 L190 L211 L213 | L110 L130 L156 L190 L210 L211 | L110 L111 L130 L137 L156 L189 | L124 L127 L134 L141 L196 A52 L197 | L117 L125 L137 L188 A50 L189 | L124 L127 L197 L204 L205 | L103 L138 L166 L224 L225 | L124 L197 L203 L205 | L103 L138 L197 L224 L225 | L114 L124 L149 L197 L202 L203 | L147 L160 L169 L207 L209 | L106 L114 L124 L126 L132 L146 L149 L197 | L147 L160 L188 L207 L209 | L109 L124 L132 L146 L197 L200 L201 | L102 L103 L162 L222 L223 | L109 L124 L197 L199 L201 | L106 L126 L132 L197 | L102 L103 L197 L222 L223 | L124 L150 L197 L198 L199 | L104 L105 L124 A49 L188 L197 | L105 L118 L124 L145 L150 | L104 L118 L150 L197 | A33 | A38 | A39 | A40 | A42 | A43 | A44 | A48 makes body 2
extrude "Extrude11" add sketch "Sketch1" against normal blind 1 contours A33 | A38 | A39 | A40 | A42 | A43 | A44 | A48 bodies 2
extrude "Extrude12" add sketch "Sketch1" against normal blind 2 contours L156 L194 L219 L221 | L183 L194 L219 L221 | L156 L192 L215 L217 | L180 L183 L219 L221 | L177 L192 L215 L217 | L175 L177 L215 L217 | L110 L156 L190 L211 L213 | L171 L173 L211 L213 | L173 L190 L211 L213 | L103 L138 L166 L224 L225 | L124 L197 L203 L205 | L103 L138 L197 L224 L225 | L147 L160 L169 L207 L209 | L147 L160 L188 L207 L209 | L102 L103 L162 L222 L223 | L109 L124 L197 L199 L201 | L102 L103 L197 L222 L223 bodies 2
extrude "Extrude13" add 4 faces at (-109.366, -27.3333, -2) (-92.6333, -28.4167, -2) (-70.6333, -27.3333, -2) (-92.6333, 28.3333, -2) along direction (0, 0, -1) blind 1 on bodies 2 bodies 2
extrude "Extrude14" add 4 faces at (2.6667, 27.1667, 2.5) (-19.3333, -28.4167, 2.5) (-2.6667, -27.3333, 2.5) (19.3333, -27.3333, 2.5) along direction (0, 0, 1) blind 1 on bodies 1 bodies 1
sketch "Sketch2" plane through (0, 0, 10.5) normal (0, 0, 1) x (-1, 0, 0)
  circle A0 centre (33.75, -22) radius 1.75
  circle A1 centre (33.75, -22) radius 1
  circle A2 centre (-33.75, -22) radius 1
  circle A3 centre (-33.75, -22) radius 1.75
  circle A4 centre (33.75, 22) radius 1
  circle A5 centre (-33.75, 22) radius 1
  circle A6 centre (-33.75, 22) radius 1.75
  circle A7 centre (33.75, 22) radius 1.75
  dimension "d168" = 2
  dimension "d169" = 2
  dimension "d170" = 2
  dimension "d171" = 2
  constraint concentric A0 A1
  constraint concentric A2 A3
  constraint concentric A5 A6
  constraint concentric A4 A7
  measures "d168" diameter of A1
  measures "d169" diameter of A2
  measures "d170" diameter of A4
  measures "d171" diameter of A5
extrude "Extrude15" cut sketch "Sketch2" against normal blind 5 contours A1 | A2 | A4 | A5 bodies 1
copy_body "Body->Comp1" bodies 2 removing the originals makes body 3 in component "Component"
copy_body "Body->Comp2" bodies 1 removing the originals makes body 4 in component "Component'"
fillet "Fillet1" radius 1 12 edges at (8, 27.75, 3.5) (24.45, 27.75, 1.5) (30, -27.875, 3.5) (8, -27.875, 3.5) (-14, -27.875, 3.5) (-38.25, 10, 0.5) (14, -27.875, 3.5) (-8, -27.875, 3.5) (-30, -27.875, 3.5) (-8, 27.75, 3.5) (18.45, 27.75, 1.5) (-38.25, 2, 0.5) on bodies 4 in component "Component'"
chamfer "Chamfer1" distance 1 angle 45 22 edges at (-39, 0, -1) (-38.4142, 28.9142, -1) (0, 29.5, -1) (38.4142, 28.9142, -1) (39, 0, -1) (38.4142, -28.9142, -1) (0, -29.5, -1) (-38.4142, -28.9142, -1) (-39, -12.75, 14.5) (-38.4142, -28.9142, 14.5) (-33.5, -29.5, 14.5) (-11, -29.5, 14.5) (11, -29.5, 14.5) (33.5, -29.5, 14.5) (38.4142, -28.9142, 14.5) (39, 0, 14.5) (38.4142, 28.9142, 14.5) (30.725, 29.5, 14.5) (13.225, 29.5, 14.5) (-22.5, 29.5, 14.5) (-38.4142, 28.9142, 14.5) (-39, 18.75, 14.5) on bodies 4 in component "Component'"
chamfer "Chamfer1'" distance 1 angle 45 6 edges at (-112, -29.5, 1.5) (-90, -29.5, 1.5) (-68, -29.5, 1.5) (-68.55, 29.5, 1.5) (-90, 29.5, 1.5) (-129, 6, 1.5) on bodies 3 in component "Component"
component "Component" placed x (1, 0, 0) y (0, 1, 0) z (0, 0, 1) at (90, 0, 13)
component "Component'" placed x (1, 0, 0) y (0, 1, 0) z (0, 0, 1) at (0, 0, 0)
